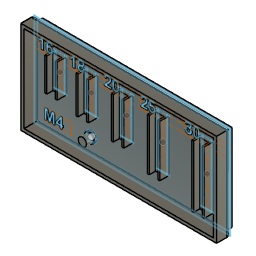
M4 Reference Caliper From 16 v5 (Autodesk Fusion 360 design; units mm, degrees)
Autodesk Fusion 360 part; units mm, degrees
note: some values were not read from the file. Chosen so that the rebuilt part matches the saved one: which bodies a step acts on; which pieces of a blend or face edit are solid.
sketch "Schizzo1" plane through (0, 0, 0) normal (0, 1, 0) x (1, 0, 0)
  line L0 (-43.0702, -51.0998) -> (51.9298, -51.0998)
  line L1 (51.9298, -51.0998) -> (51.9298, -6.0998)
  line L2 (51.9298, -6.0998) -> (-43.0702, -6.0998)
  line L3 (-43.0702, -6.0998) -> (-43.0702, -51.0998)
  line L4 (-40.8542, -38.0712) -> (-36.5648, -38.0712) construction
  line L5 (-36.5648, -38.0712) -> (-36.5648, -43.6885) construction
  line L6 (-36.5648, -43.6885) -> (-40.8542, -43.6885) construction
  line L7 (-40.8542, -43.6885) -> (-40.8542, -38.0712) construction
  line L8 (-25.562, -38.0712) -> (-21.5729, -38.0712) construction
  line L9 (-21.5729, -38.0712) -> (-21.5729, -43.6885) construction
  line L10 (-21.5729, -43.6885) -> (-25.562, -43.6885) construction
  line L11 (-25.562, -43.6885) -> (-25.562, -38.0712) construction
  line L12 (-9.0963, -38.0712) -> (-1.5386, -38.0712) construction
  line L13 (-1.5386, -38.0712) -> (-1.5386, -43.6885) construction
  line L14 (-1.5386, -43.6885) -> (-9.0963, -43.6885) construction
  line L15 (-9.0963, -43.6885) -> (-9.0963, -38.0712) construction
  line L16 (8.5895, -38.0712) -> (15.2292, -38.0712) construction
  line L17 (15.2292, -38.0712) -> (15.2292, -43.6885) construction
  line L18 (15.2292, -43.6885) -> (8.5895, -43.6885) construction
  line L19 (8.5895, -43.6885) -> (8.5895, -38.0712) construction
  line L20 (30.1881, -38.0712) -> (37.6297, -38.0712) construction
  line L21 (37.6297, -38.0712) -> (37.6297, -43.6885) construction
  line L22 (37.6297, -43.6885) -> (30.1881, -43.6885) construction
  line L23 (30.1881, -43.6885) -> (30.1881, -38.0712) construction
  line L24 (-33.428, -41.5998) -> (-27.428, -41.5998)
  line L25 (-27.428, -41.5998) -> (-27.428, -25.5998)
  line L26 (-27.428, -25.5998) -> (-33.428, -25.5998)
  line L27 (-33.428, -25.5998) -> (-33.428, -41.5998)
  line L28 (-30.428, -41.5998) -> (-30.428, -25.5998) construction
  line L29 (-28.328, -25.5998) -> (-32.528, -25.5998)
  line L30 (-32.528, -25.5998) -> (-32.528, -41.5998)
  line L31 (-32.528, -41.5998) -> (-28.328, -41.5998)
  line L32 (-28.328, -41.5998) -> (-28.328, -25.5998)
  line L33 (-28.328, -25.5998) -> (-32.528, -41.5998) construction
  line L34 (-32.528, -25.5998) -> (-28.328, -41.5998) construction
  line L35 (-12.2933, -23.5998) -> (-18.2933, -23.5998)
  line L36 (-17.3933, -23.5998) -> (-13.1933, -41.5998) construction
  line L37 (-13.1933, -23.5998) -> (-17.3933, -23.5998)
  line L38 (-13.1933, -41.5998) -> (-13.1933, -23.5998)
  line L39 (-17.3933, -23.5998) -> (-17.3933, -41.5998)
  line L40 (-13.1933, -23.5998) -> (-17.3933, -41.5998) construction
  line L41 (-15.2933, -41.5998) -> (-15.2933, -23.5998) construction
  line L42 (-18.2933, -41.5998) -> (-12.2933, -41.5998)
  line L43 (-18.2933, -23.5998) -> (-18.2933, -41.5998)
  line L44 (-12.2933, -41.5998) -> (-12.2933, -23.5998)
  line L45 (-17.3933, -41.5998) -> (-13.1933, -41.5998)
  line L46 (3.9863, -41.5998) -> (3.9863, -21.5998)
  line L47 (-1.1137, -21.5998) -> (-1.1137, -41.5998)
  line L48 (4.8863, -41.5998) -> (4.8863, -21.5998)
  line L49 (-1.1137, -41.5998) -> (4.8863, -41.5998)
  line L50 (3.9863, -21.5998) -> (-0.2137, -41.5998) construction
  line L51 (3.9863, -21.5998) -> (-0.2137, -21.5998)
  line L52 (-0.2137, -21.5998) -> (-0.2137, -41.5998)
  line L53 (-0.2137, -21.5998) -> (3.9863, -41.5998) construction
  line L54 (4.8863, -21.5998) -> (-1.1137, -21.5998)
  line L55 (1.8863, -41.5998) -> (1.8863, -21.5998) construction
  line L56 (-0.2137, -41.5998) -> (3.9863, -41.5998)
  line L57 (17.2557, -41.5998) -> (21.4557, -41.5998)
  line L58 (17.2557, -16.5998) -> (17.2557, -41.5998)
  line L59 (16.3557, -41.5998) -> (22.3557, -41.5998)
  line L60 (21.4557, -41.5998) -> (21.4557, -16.5998)
  line L61 (21.4557, -16.5998) -> (17.2557, -41.5998) construction
  line L62 (22.3557, -16.5998) -> (16.3557, -16.5998)
  line L63 (19.3557, -41.5998) -> (19.3557, -16.5998) construction
  line L64 (16.3557, -16.5998) -> (16.3557, -41.5998)
  line L65 (21.4557, -16.5998) -> (17.2557, -16.5998)
  line L66 (17.2557, -16.5998) -> (21.4557, -41.5998) construction
  line L67 (22.3557, -41.5998) -> (22.3557, -16.5998)
  line L68 (-43.0702, -41.5998) -> (51.9298, -41.5998) construction
  line L69 (37.9229, -41.5998) -> (43.9229, -41.5998)
  line L70 (43.0229, -11.5998) -> (38.8229, -41.5998) construction
  line L71 (43.9229, -41.5998) -> (43.9229, -11.5998)
  line L72 (37.9229, -11.5998) -> (37.9229, -41.5998)
  line L73 (43.0229, -41.5998) -> (43.0229, -11.5998)
  line L74 (43.0229, -11.5998) -> (38.8229, -11.5998)
  line L75 (40.9229, -41.5998) -> (40.9229, -11.5998) construction
  line L76 (38.8229, -11.5998) -> (38.8229, -41.5998)
  line L77 (38.8229, -41.5998) -> (43.0229, -41.5998)
  line L78 (38.8229, -11.5998) -> (43.0229, -41.5998) construction
  line L79 (43.9229, -11.5998) -> (37.9229, -11.5998)
  line L80 (-43.0702, -43.6885) -> (51.9298, -43.6885) construction
  line L81 (50.4298, -49.5998) -> (50.4298, -7.5998)
  line L82 (50.4298, -7.5998) -> (-41.5702, -7.5998)
  line L83 (-41.5702, -7.5998) -> (-41.5702, -49.5998)
  line L84 (-41.5702, -49.5998) -> (50.4298, -49.5998)
  line L85 (-38, -10) -> (-25, -10) construction
  line L86 (-25, -10) -> (-25, -15) construction
  line L87 (-25, -15) -> (-38, -15) construction
  line L88 (-38, -15) -> (-38, -10) construction
  line L89 (-43.0702, -38.0712) -> (50.4298, -38.0712) construction
  circle A0 centre (-15.227, -14.1775) radius 2
  circle A1 centre (-15.227, -14.1775) radius 2.5
  point P0 (-30.428, -33.5998)
  point P1 (-15.2933, -32.5998)
  point P2 (1.8863, -31.5998)
  point P3 (19.3557, -29.0998)
  point P4 (40.9229, -26.5998)
  dimension "d1" = 45
  dimension "d2" = 5
  dimension "d3" = 5
  dimension "d4" = 5
  dimension "d5" = 5
  dimension "d6" = 5
  dimension "d7" = 6
  dimension "d8" = 16
  dimension "d9" = 4.2
  dimension "d21" = 6
  dimension "d22" = 18
  dimension "d23" = 4.2
  dimension "d24" = 6
  dimension "d25" = 20
  dimension "d26" = 4.2
  dimension "d27" = 6
  dimension "d28" = 25
  dimension "d29" = 4.2
  dimension "d30" = 6
  dimension "d31" = 30
  dimension "d32" = 4.2
  dimension "d33" = 95
  dimension "d34" = -1.5
  dimension "d37" = 5
  dimension "d40" = 4
  dimension "d41" = 5
  dimension "d50" = 8
  text T0 "16" font "Arial" height 5 bold align left top in box 4.2894 x 5.6173 at (-40.8542, -38.0712) x (1, 0) y (0, -1) spacing 1
  text T1 "18" font "Arial" height 5 bold align left top in box 3.9891 x 5.6173 at (-25.562, -38.0712) x (1, 0) y (0, -1) spacing 1
  text T2 "20" font "Arial" height 5 bold align left top in box 7.5577 x 5.6173 at (-9.0963, -38.0712) x (1, 0) y (0, -1) spacing 1
  text T3 "25" font "Arial" height 5 bold align left top in box 6.6397 x 5.6173 at (8.5895, -38.0712) x (1, 0) y (0, -1) spacing 1
  text T4 "30" font "Arial" height 5 bold align left top in box 7.4417 x 5.6173 at (30.1881, -38.0712) x (1, 0) y (0, -1) spacing 1
  text T5 "M4" font "Arial" height 5 bold align left top in box 13 x 5 at (-38, -10) x (1, 0) y (0, -1) spacing 1
  constraint horizontal L0
  constraint vertical L1
  constraint horizontal L2
  constraint vertical L3
  constraint horizontal L24
  constraint vertical L25
  constraint horizontal L26
  constraint vertical L27
  constraint midpoint L24 L28.start
  constraint midpoint L26 L28.end
  constraint horizontal L29
  constraint perpendicular L29 L30
  constraint parallel L29 L31
  constraint parallel L30 L32
  constraint coincident L33 P0
  constraint coincident L34 P0
  constraint coincident L26 L29.start
  constraint midpoint L28 P0
  constraint horizontal L42
  constraint vertical L44
  constraint horizontal L35
  constraint vertical L43
  constraint midpoint L41.start L42
  constraint midpoint L41.end L35
  constraint horizontal L37
  constraint perpendicular L37 L39
  constraint parallel L37 L45
  constraint parallel L38 L39
  constraint coincident P1 L40
  constraint coincident P1 L36
  constraint coincident L37.start L35
  constraint midpoint P1 L41
  constraint horizontal L49
  constraint vertical L48
  constraint horizontal L54
  constraint vertical L47
  constraint midpoint L55.start L49
  constraint midpoint L55.end L54
  constraint horizontal L51
  constraint perpendicular L51 L52
  constraint parallel L51 L56
  constraint parallel L46 L52
  constraint coincident P2 L50
  constraint coincident P2 L53
  constraint coincident L46.end L54
  constraint midpoint P2 L55
  constraint horizontal L59
  constraint vertical L67
  constraint horizontal L62
  constraint vertical L64
  constraint midpoint L63.start L59
  constraint midpoint L63.end L62
  constraint horizontal L65
  constraint perpendicular L58 L65
  constraint parallel L57 L65
  constraint parallel L58 L60
  constraint coincident P3 L61
  constraint coincident P3 L66
  constraint coincident L60.end L62
  constraint midpoint P3 L63
  constraint coincident L3 L68.start
  constraint coincident L1 L68.end
  constraint perpendicular L1 L68
  constraint collinear L31 L68
  constraint collinear L49 L68
  constraint collinear L59 L68
  constraint horizontal L69
  constraint vertical L71
  constraint horizontal L79
  constraint vertical L72
  constraint midpoint L75.start L69
  constraint midpoint L75.end L79
  constraint horizontal L74
  constraint perpendicular L74 L76
  constraint parallel L74 L77
  constraint parallel L73 L76
  constraint coincident P4 L70
  constraint coincident P4 L78
  constraint coincident L70.start L79
  constraint midpoint P4 L75
  constraint coincident L3 L80.start
  constraint coincident L1 L80.end
  constraint perpendicular L1 L80
  constraint collinear L42 L68
  constraint collinear L68 L69
  constraint collinear L6 L80
  constraint collinear L10 L80
  constraint collinear L14 L80
  constraint collinear L18 L80
  constraint collinear L22 L80
  constraint coincident L3 L89.start
  constraint coincident L81 L89.end
  constraint perpendicular L81 L89
  constraint collinear L4 L89
  constraint collinear L8 L89
  constraint collinear L12 L89
  constraint collinear L16 L89
  constraint collinear L20 L89
  constraint concentric A0 A1
  measures "d1" distance of L0 L2
  measures "d7" distance of L24.start L24.end
  measures "d8" distance of L24.start L26.end
  measures "d9" distance of L30 L32
  measures "d21" distance of L42.start L42.end
  measures "d22" distance of L42.start L35.end
  measures "d23" distance of L38 L39
  measures "d24" distance of L47.end L48.start
  measures "d25" distance of L47.start L47.end
  measures "d26" distance of L46 L52
  measures "d27" distance of L59.end L59.start
  measures "d28" distance of L62.end L59.start
  measures "d29" distance of L58 L60
  measures "d30" distance of L69.start L69.end
  measures "d31" distance of L69.start L72.start
  measures "d32" distance of L73 L76
  measures "d33" distance of L1 L3
  measures "d40" diameter of A0
  measures "d41" diameter of A1
  measures "d50" distance of L68 L84
extrude "Estrusione1" add sketch "Schizzo1" along normal blind 0.4 text T0 T1 T2 T3 T4 T5 makes body 1 at (-38.9772, 0, 41.5659) makes body 2 at (32.1705, 0, 41.3816) makes body 3 at (-7.491, 0, 38.9852) makes body 4 at (13.2461, 0, 42.1707) makes body 5 at (10.1948, 0, 38.9852) makes body 6 at (-19.8912, 0, 41.369) makes body 7 at (-29.8815, 0, 13.4754) makes body 8 at (-37.6874, 0, 12.9786) makes body 9 at (-36.5108, 0, 41.1495) makes body 10 at (-23.685, 0, 41.5659) makes body 11 at (37.0059, 0, 40.7994) makes body 12 at (-2.1898, 0, 40.7994)
extrude "Estrusione2" add sketch "Schizzo1" along normal blind 0.5 separate body contours L0 L1 L2 L3 | L24 L26 L27 L30 | L24 L26 L29 L30 L31 L32 | L24 L25 L26 L32 | L35 L38 L42 L44 | L35 L37 L38 L39 L42 L45 | L35 L39 L42 L43 | L46 L49 L51 L52 L54 L56 | L46 L48 L49 L54 | L47 L49 L52 L54 | L57 L58 L59 L60 L62 L65 | L58 L59 L62 L64 | L59 L60 L62 L67 | L69 L72 L76 L79 | L69 L73 L74 L76 L77 L79 | L69 L71 L73 L79 | L81 L82 L83 L84 | A0 | A1 makes body 13
extrude "Estrusione7" cut sketch "Schizzo1" along normal blind 0.4 text T0 T1 T2 T3 T5 T4 bodies 13
extrude "Estrusione6" add sketch "Schizzo1" against normal blind 6.5 contours L0 L1 L2 L3 bodies 13
extrude "Estrusione4" add sketch "Schizzo1" against normal blind 4.5 contours L24 L26 L27 L30 | L24 L26 L29 L30 L31 L32 | L24 L25 L26 L32 | L35 L38 L42 L44 | L35 L37 L38 L39 L42 L45 | L35 L39 L42 L43 | L46 L49 L51 L52 L54 L56 | L46 L48 L49 L54 | L47 L49 L52 L54 | L57 L58 L59 L60 L62 L65 | L58 L59 L62 L64 | L59 L60 L62 L67 | L69 L72 L76 L79 | L69 L73 L74 L76 L77 L79 | L69 L71 L73 L79 | A0 bodies 13
extrude "Estrusione8" add sketch "Schizzo1" against normal blind 1 contours A1 bodies 13
extrude "Estrusione5" cut sketch "Schizzo1" along normal blind 3 from surface at -4.5 contours L24 L26 L29 L30 L31 L32 | L35 L37 L38 L39 L42 L45 | L46 L49 L51 L52 L54 L56 | L57 L58 L59 L60 L62 L65 | L69 L73 L74 L76 L77 L79 bodies 13
sketch "Schizzo2" plane through (0, 0.5, 0) normal (0, 1, 0) x (-1, 0, 0)
  line L0 (43.0702, 6.0998) -> (43.0702, 51.0998)
  line L1 (43.0702, 51.0998) -> (-51.9298, 51.0998)
  line L2 (-51.9298, 51.0998) -> (-51.9298, 6.0998)
  line L3 (-51.9298, 6.0998) -> (43.0702, 6.0998)
  line L4 (-51.9298, 51.0998) -> (43.0702, 51.0998) construction
  line L5 (43.0702, 51.0998) -> (43.0702, 6.0998) construction
  line L6 (43.0702, 6.0998) -> (-51.9298, 6.0998) construction
  line L7 (-51.9298, 6.0998) -> (-51.9298, 51.0998) construction
  line L8 (43.0702, 51.0998) -> (-51.9298, 51.0998) construction
  line L9 (-51.9298, 51.0998) -> (-51.9298, 6.0998) construction
  line L10 (-51.9298, 6.0998) -> (43.0702, 6.0998) construction
  line L11 (43.0702, 6.0998) -> (43.0702, 51.0998) construction
  line L12 (-51.9298, 28.5998) -> (-50, 28.5998) construction
  line L13 (-50, 28.5998) -> (43.0702, 28.5998) construction
  line L14 (-4.4298, 51.0998) -> (-4.4298, 6.0998) construction
  line L15 (41.5702, 7.5998) -> (-50.4298, 7.5998)
  line L16 (-50.4298, 7.5998) -> (-50.4298, 49.5998)
  line L17 (-50.4298, 49.5998) -> (41.5702, 49.5998)
  line L18 (41.5702, 49.5998) -> (41.5702, 7.5998)
  line L19 (41.5702, 7.5998) -> (-50.4298, 49.5998) construction
  line L20 (-50.4298, 7.5998) -> (41.5702, 49.5998) construction
  point P0 (-4.4298, 28.5998)
  dimension "d44" = 1.5
  dimension "d45" = 1.5
  constraint horizontal L4
  constraint vertical L5
  constraint horizontal L6
  constraint vertical L7
  constraint collinear L4 L8
  constraint collinear L7 L9
  constraint collinear L6 L10
  constraint collinear L5 L11
  constraint midpoint L9 L12.start
  constraint perpendicular L9 L12
  constraint midpoint L11 L13.end
  constraint perpendicular L11 L13
  constraint midpoint L4 L14.start
  constraint midpoint L6 L14.end
  constraint horizontal L15
  constraint perpendicular L15 L16
  constraint parallel L15 L17
  constraint parallel L16 L18
  constraint coincident L19 P0
  constraint coincident L20 P0
  constraint midpoint L14 P0
  measures "d44" distance of L7 L16
  measures "d45" distance of L4 L17
extrude "Estrusione9" add sketch "Schizzo2" along normal blind 2 contours L15 L16 L17 L18 bodies 13
fillet "Raccordo1" radius 2 4 edges at (4.4298, 0.5, 6.0998) (51.9298, 0.5, 28.5998) (-43.0702, 0.5, 28.5998) (4.4298, 0.5, 51.0998) on bodies 13
equation "d21 = d7"
equation "d23 = d9"
equation "d24 = d7"
equation "d26 = d9"
equation "d27 = d7"
equation "d29 = d9"
equation "d30 = d7"
equation "d32 = d9"
equation "d41 = d40 + 1 mm"
equation "d45 = d44"
